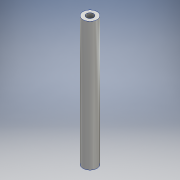
# Autodesk Inventor part: スペーサーm3-55
Saved by Autodesk Inventor 2020.2 (Build 242310000, 310)
## iProperties
Created: 2016-10-20
Part Number: スペーサーm3-55
Material: アルミニウム 2014-T4
Document SubType Name: Modeling
Designer: Takumi
Density: 2.8 g/cm^3
Appearance: アルミニウム - フラット
Author: Takumi
Autodesk Inventor part; units mm, degrees
ref_plane "YZ Plane" through (0, 0, 0) normal (1, 0, 0) x (0, 1, 0)
ref_plane "XZ Plane" through (0, 0, 0) normal (0, 1, 0) x (-1, 0, 0)
ref_plane "XY Plane" through (0, 0, 0) normal (0, 0, 1) x (1, 0, 0)
sketch "スケッチ1" plane through (0, 0, 0) normal (0, 0, 1) x (1, 0, 0)
  circle A0 centre (0, 0) radius 3
  dimension "d0" = 6
  constraints: 1 centre point, 1 coincident
  measures "d0" diameter of A0
extrude "押し出し1" add sketch "スケッチ1" along normal blind 55
sketch "スケッチ2" plane through (0, 0, 55) normal (0, 0, 1) x (1, 0, 0)
  circle A0 centre (0, 0) radius 1.5
  dimension "d3" = 3
  constraints: 1 centre point, 1 coincident
  measures "d3" diameter of A0
extrude "押し出し2" cut sketch "スケッチ2" against normal blind 6
sketch "スケッチ3" plane through (0, 0, 0) normal (0, 0, -1) x (-1, 0, 0)
  circle A0 centre (0, 0) radius 1.5 projected
  circle A1 centre (0, 0) radius 1.5
  dimension "d6" = 3
  constraints: 1 centre point, 1 coincident
  measures "d6" diameter of A1
extrude "押し出し3" cut sketch "スケッチ3" against normal blind 6
